Autodesk Fusion 360 part; units mm, degrees
(part 2 of 2)
  line L917 (-904.3735, -2837.0745) -> (-14000, -2837.0745)
  line L918 (-1204.3735, -11252.1545) -> (-1204.3735, -3137.0745)
  line L919 (-1204.3735, -3137.0745) -> (-14000, -3137.0745)
  line L920 (-14000, -3137.0745) -> (-14000, -2837.0745)
  line L921 (-1204.3735, -11252.1545) -> (-904.3735, -11252.1545)
  line L922 (-7006.0828, -10336.1218) -> (-8698.4144, -10336.1218)
  line L923 (-8698.4144, -10336.1218) -> (-8698.4144, -3137.0745)
  line L924 (-8698.4144, -3137.0745) -> (-7006.0828, -3137.0745)
  line L925 (-7006.0828, -3137.0745) -> (-7006.0828, -10336.1218)
  line L926 (-5639.7967, -10336.1218) -> (-1204.3735, -10336.1218)
  line L927 (-1204.3735, -10336.1218) -> (-1204.3735, -10036.1218)
  line L928 (-1204.3735, -10036.1218) -> (-5639.7967, -10036.1218)
  line L929 (-5639.7967, -10036.1218) -> (-5639.7967, -10336.1218)
  line L930 (-14200, -10000) -> (-9900, -10000)
  line L931 (-9900, -10000) -> (-9900, -10300)
  line L932 (-9900, -10300) -> (-14200, -10300)
  line L933 (-14200, -10300) -> (-14200, -10000)
  line L934 (-1060.2048, -1766.9819) -> (-14240.8305, -1766.9819)
  line L935 (-14240.8305, 3555.5601) -> (-1060.2048, 3555.5601)
  line L936 (-1360.2048, -1466.9819) -> (-13940.8305, -1466.9819)
  line L937 (-13940.8305, 3255.5601) -> (-1360.2048, 3255.5601)
  line L938 (-8963.6202, 3255.5601) -> (-9263.6202, 3255.5601)
  line L939 (-9263.6202, 3255.5601) -> (-9263.6202, -1466.9819)
  line L940 (-9263.6202, -1466.9819) -> (-8963.6202, -1466.9819)
  line L941 (-8963.6202, -1466.9819) -> (-8963.6202, 3255.5601)
  line L942 (-13940.8305, 758.7969) -> (-9263.6202, 758.7969)
  line L943 (-9263.6202, 758.7969) -> (-9263.6202, 1058.7969)
  line L944 (-9263.6202, 1058.7969) -> (-13940.8305, 1058.7969)
  line L945 (-13940.8305, 1058.7969) -> (-13940.8305, 758.7969)
  line L946 (-13940.8305, 1674.4472) -> (-14240.8305, 1674.4472)
  line L947 (-14240.8305, 201.9825) -> (-13940.8305, 201.9825)
  line L948 (-13940.8305, 758.7969) -> (-13940.8305, 1058.7969)
  line L949 (-1360.2048, 2862.3179) -> (-1060.2048, 2862.3179)
  line L950 (-1060.2048, 1785.8101) -> (-1360.2048, 1785.8101)
  line L951 (-1060.2048, 3555.5601) -> (-1060.2048, 2862.3179)
  line L952 (-1060.2048, 1785.8101) -> (-1060.2048, -1766.9819)
  line L953 (-1360.2048, 3255.5601) -> (-1360.2048, 2862.3179)
  line L954 (-1360.2048, 1785.8101) -> (-1360.2048, -1466.9819)
  line L955 (-14240.8305, -1766.9819) -> (-14240.8305, 201.9825)
  line L956 (-14240.8305, 1674.4472) -> (-14240.8305, 3555.5601)
  line L957 (-13940.8305, 1674.4472) -> (-13940.8305, 3255.5601)
  line L958 (-13940.8305, -1466.9819) -> (-13940.8305, 201.9825)
  line L959 (-13940.8305, 758.7969) -> (-13940.8305, 1058.7969)
  line L960 (-14240.8305, 3555.5601) -> (-13940.8305, 3555.5601)
  line L961 (-13940.8305, 3555.5601) -> (-13940.8305, 6300)
  line L962 (-13940.8305, 6300) -> (-14240.8305, 6300)
  line L963 (-14240.8305, 6300) -> (-14240.8305, 3555.5601)
  line L964 (-13500, 6000) -> (-11400, 6000)
  line L965 (-11400, 6000) -> (-11400, 3555.5601)
  line L966 (-13500, 6300) -> (-11100, 6300)
  line L967 (-11100, 6300) -> (-11100, 3555.5601)
  line L968 (-13500, 6000) -> (-13500, 6300)
  line L969 (-10700, 6000) -> (-9300, 6000)
  line L970 (-9300, 6000) -> (-9300, 3555.5601)
  line L971 (-10700, 6300) -> (-9000, 6300)
  line L972 (-9000, 6300) -> (-9000, 3555.5601)
  line L973 (-10700, 6300) -> (-10700, 6000)
  line L974 (-14200, 10200) -> (-9100, 10200)
  line L975 (-9100, 10200) -> (-9100, 7400)
  line L976 (-14200, 7400) -> (-14200, 10200)
  line L977 (-13900, 7700) -> (-13900, 9900)
  line L978 (-13900, 9900) -> (-9400, 9900)
  line L979 (-9400, 9900) -> (-9400, 7700)
  line L980 (-12500, 7700) -> (-12500, 7400)
  line L981 (-12000, 7400) -> (-12000, 7700)
  line L982 (-9800, 7700) -> (-9800, 7400)
  line L983 (-9400, 7400) -> (-9400, 7700)
  line L984 (-12000, 9900) -> (-11700, 9900)
  line L985 (-11700, 9900) -> (-11700, 7700)
  line L986 (-11700, 7700) -> (-12000, 7700)
  line L987 (-12000, 7700) -> (-12000, 9900)
  line L988 (-12500, 7400) -> (-14200, 7400)
  line L989 (-9800, 7700) -> (-12000, 7700)
  line L990 (-12500, 7700) -> (-13900, 7700)
  line L991 (-9100, 7400) -> (-9400, 7400)
  line L992 (-9800, 7400) -> (-12000, 7400)
  line L993 (-12500, 12200) -> (-13900, 12200)
  line L994 (-13900, 12200) -> (-13900, 14100)
  line L995 (-13900, 14100) -> (-12100, 14100)
  line L996 (-12100, 14100) -> (-12100, 12100)
  line L997 (-12500, 11900) -> (-14200, 11900)
  line L998 (-14200, 11900) -> (-14200, 14400)
  line L999 (-14200, 14400) -> (-11800, 14400)
  line L1000 (-11800, 14400) -> (-11800, 12200)
  line L1001 (-12500, 12200) -> (-12500, 11900)
  line L1002 (-12100, 12100) -> (-12100, 11900)
  line L1003 (-12100, 11900) -> (-9800, 11900)
  line L1004 (-9800, 11900) -> (-9800, 12200)
  line L1005 (-9800, 12200) -> (-11800, 12200)
  line L1006 (-11800, 14100) -> (-9400, 14100)
  line L1007 (-9400, 14100) -> (-9400, 12100)
  line L1008 (-9400, 12100) -> (-9100, 12100)
  line L1009 (-9100, 12100) -> (-9100, 14100)
  line L1010 (-11800, 14400) -> (-1049.606, 14400)
  line L1011 (-1049.606, 14400) -> (-1060.2048, 3555.5601)
  line L1012 (-9100, 14100) -> (-1595.3922, 14100)
  line L1013 (-1360.2048, 3555.5601) -> (-1360.2048, 14100)
  line L1014 (-1360.2048, 14100) -> (-1595.3922, 14100)
  line L1015 (-39100, 9500) -> (-31300, 9500)
  line L1016 (-31300, 9500) -> (-31300, 14500)
  line L1017 (-31300, 14500) -> (-27900, 14500)
  line L1018 (-39100, 9200) -> (-31000, 9200)
  line L1019 (-31000, 9200) -> (-31000, 14200)
  line L1020 (-31000, 14200) -> (-27900, 14200)
  line L1021 (-27900, 14500) -> (-27900, 14200)
  line L1022 (-31000, 9500) -> (-22000, 9500)
  line L1023 (-22000, 9500) -> (-22000, 14000)
  line L1024 (-22000, 14000) -> (-25200, 14000)
  line L1025 (-31000, 9200) -> (-21700, 9200)
  line L1026 (-21700, 9200) -> (-21700, 14300)
  line L1027 (-21700, 14300) -> (-25200, 14300)
  line L1028 (-25200, 14300) -> (-25200, 14000)
  line L1029 (-21700, 14300) -> (-18691.9492, 14300)
  line L1030 (-18691.9492, 14300) -> (-18691.9492, 14000)
  line L1031 (-18691.9492, 14000) -> (-21700, 14000)
  line L1032 (-26700, 14400) -> (-26400, 14400)
  line L1033 (-26400, 14400) -> (-26400, 9500)
  line L1034 (-26400, 9500) -> (-26700, 9500)
  line L1035 (-26700, 9500) -> (-26700, 14400)
  line L1036 (-21700, 9200) -> (-17491.9492, 9200)
  line L1037 (-17491.9492, 9200) -> (-17491.9492, 8300)
  line L1038 (-17491.9492, 8300) -> (-17191.9492, 8300)
  line L1039 (-17191.9492, 8300) -> (-17191.9492, 14200)
  line L1040 (-17191.9492, 9500) -> (-17191.9492, 8600)
  line L1041 (-21700, 9500) -> (-17491.9492, 9500)
  line L1042 (-17491.9492, 9500) -> (-17491.9492, 14200)
  line L1043 (-17491.9492, 14200) -> (-17191.9492, 14200)
  line L1044 (-31410.3645, 9200) -> (-31410.3645, 3640.3591)
  line L1045 (-31410.3645, 3640.3591) -> (-17160.8557, 3640.3591)
  line L1046 (-17160.8557, 3640.3591) -> (-17160.8557, 6838.9487)
  line L1047 (-31110.3645, 9200) -> (-31110.3645, 3940.3591)
  line L1048 (-31110.3645, 3940.3591) -> (-17460.8557, 3940.3591)
  line L1049 (-17460.8557, 3940.3591) -> (-17460.8557, 6838.9487)
  line L1050 (-17160.8557, 6838.9487) -> (-17460.8557, 6838.9487)
  line L1051 (15034.8266, -18499.5167) -> (15034.8266, -18199.5167)
  dimension "d1" = 90
  dimension "d4" = 90
  dimension "d13" = 90
  dimension "d24" = 90
  dimension "d25" = 90
  dimension "d68" = 90
  dimension "d101" = 90
  constraint horizontal L0
  constraint perpendicular L1 L2
  constraint perpendicular L2 L3
  constraint perpendicular L3 L4
  constraint perpendicular L2 L5
  constraint perpendicular L5 L6
  constraint perpendicular L6 L7
  constraint perpendicular L0 L16
  constraint perpendicular L16 L17
  constraint perpendicular L17 L18
  constraint perpendicular L18 L19
  constraint perpendicular L19 L20
  constraint perpendicular L18 L21
  constraint perpendicular L21 L22
  constraint perpendicular L22 L23
  constraint vertical L24
  constraint perpendicular L25 L26
  constraint perpendicular L26 L27
  constraint perpendicular L25 L28
  constraint perpendicular L28 L29
  constraint perpendicular L29 L30
  constraint vertical L52
  constraint coincident L38 L52.end
  constraint coincident L38 L53.start
  constraint perpendicular L38 L53
  constraint parallel L18 L31
  constraint parallel L22 L32
  constraint parallel L30 L33
  constraint parallel L29 L34
  constraint parallel L27 L35
  constraint parallel L26 L36
  constraint parallel L25 L37
  constraint parallel L24 L38
  constraint parallel L21 L39
  constraint parallel L20 L40
  constraint parallel L19 L41
  constraint parallel L16 L42
  constraint parallel L0 L43
  constraint parallel L1 L44
  constraint parallel L2 L45
  constraint parallel L3 L46
  constraint parallel L4 L47
  constraint parallel L5 L48
  constraint parallel L6 L49
  constraint parallel L7 L50
  constraint horizontal L55
  constraint vertical L56
  constraint horizontal L57
  constraint vertical L58
  constraint coincident L38 L55.start
  constraint horizontal L59
  constraint vertical L60
  constraint horizontal L61
  constraint vertical L62
  constraint coincident L36 L60.end
  constraint perpendicular L63 L66
  constraint perpendicular L66 L67
  constraint coincident L63 L68.end
  constraint perpendicular L63 L68
  constraint horizontal L69
  constraint vertical L70
  constraint horizontal L71
  constraint vertical L72
  constraint coincident L38 L70.end
  constraint coincident L38 L73.start
  constraint perpendicular L38 L73
  constraint perpendicular L73 L74
  constraint perpendicular L38 L75
  constraint perpendicular L75 L76
  constraint perpendicular L76 L80
  constraint coincident L36 L81.start
  constraint perpendicular L36 L81
  constraint perpendicular L81 L82
  constraint perpendicular L36 L83
  constraint perpendicular L84 L85
  constraint perpendicular L85 L89
  constraint perpendicular L35 L90
  constraint perpendicular L36 L91
  constraint perpendicular L35 L92
  constraint perpendicular L36 L93
  constraint perpendicular L93 L94
  constraint perpendicular L93 L95
  constraint perpendicular L36 L96
  constraint coincident L35 L97.end
  constraint perpendicular L35 L97
  constraint horizontal L98
  constraint vertical L99
  constraint horizontal L100
  constraint vertical L101
  constraint coincident L35 L102.start
  constraint perpendicular L35 L102
  constraint perpendicular L102 L103
  constraint perpendicular L103 L104
  constraint perpendicular L104 L105
  constraint horizontal L110
  constraint vertical L111
  constraint horizontal L112
  constraint vertical L113
  constraint coincident L35 L111.end
  constraint coincident L35 L114.start
  constraint perpendicular L35 L114
  constraint perpendicular L114 L115
  constraint perpendicular L35 L116
  constraint perpendicular L116 L117
  constraint perpendicular L117 L121
  constraint horizontal L122
  constraint vertical L123
  constraint horizontal L124
  constraint vertical L125
  constraint coincident L35 L123.end
  constraint perpendicular L35 L126
  constraint perpendicular L35 L128
  constraint perpendicular L35 L130
  constraint parallel L134 L136
  constraint perpendicular L134 L137
  constraint perpendicular L137 L138
  constraint perpendicular L134 L139
  constraint perpendicular L139 L140
  constraint perpendicular L140 L141
  constraint perpendicular L141 L142
  constraint perpendicular L142 L143
  constraint perpendicular L143 L144
  constraint perpendicular L144 L145
  constraint perpendicular L145 L146
  constraint perpendicular L146 L147
  constraint perpendicular L34 L148
  constraint perpendicular L148 L149
  constraint vertical L150
  constraint perpendicular L150 L151
  constraint perpendicular L153 L154
  constraint perpendicular L154 L155
  constraint perpendicular L155 L156
  constraint perpendicular L164 L165
  constraint coincident L159 L166.end
  constraint perpendicular L159 L166
  constraint perpendicular L165 L167
  constraint perpendicular L167 L168
  constraint coincident L159 L169.end
  constraint perpendicular L159 L169
  constraint horizontal L170
  constraint vertical L171
  constraint horizontal L172
  constraint vertical L173
  constraint coincident L159 L171.end
  constraint vertical L174
  constraint perpendicular L174 L175
  constraint perpendicular L175 L178
  constraint horizontal L185
  constraint vertical L179
  constraint horizontal L180
  constraint vertical L181
  constraint vertical L182
  constraint horizontal L183
  constraint vertical L184
  constraint collinear L185 L186
  constraint coincident L160 L187.start
  constraint perpendicular L160 L187
  constraint perpendicular L187 L188
  constraint horizontal L192
  constraint vertical L193
  constraint horizontal L194
  constraint vertical L195
  constraint coincident L160 L193.end
  constraint coincident L160 L196.start
  constraint perpendicular L160 L196
  constraint perpendicular L196 L197
  constraint perpendicular L160 L198
  constraint perpendicular L198 L199
  constraint horizontal L204
  constraint vertical L205
  constraint horizontal L206
  constraint vertical L207
  constraint coincident L160 L205.end
  constraint coincident L160 L208.start
  constraint perpendicular L160 L208
  constraint perpendicular L208 L209
  constraint perpendicular L160 L210
  constraint perpendicular L210 L211
  constraint horizontal L216
  constraint vertical L217
  constraint horizontal L218
  constraint vertical L219
  constraint coincident L160 L220.start
  constraint perpendicular L160 L220
  constraint perpendicular L220 L221
  constraint perpendicular L221 L222
  constraint perpendicular L222 L223
  constraint perpendicular L223 L227
  constraint parallel L160 L228
  constraint coincident L160 L229.end
  constraint perpendicular L160 L229
  constraint horizontal L233
  constraint vertical L234
  constraint horizontal L235
  constraint vertical L236
  constraint coincident L160 L233.start
  constraint horizontal L237
  constraint vertical L238
  constraint horizontal L239
  constraint vertical L240
  constraint coincident L236 L237.start
  constraint vertical L241
  constraint coincident L236 L242.end
  constraint perpendicular L236 L242
  constraint perpendicular L241 L245
  constraint perpendicular L241 L246
  constraint perpendicular L246 L247
  constraint perpendicular L247 L248
  constraint perpendicular L248 L249
  constraint perpendicular L243 L250
  constraint vertical L255
  constraint coincident L253 L256.end
  constraint perpendicular L253 L256
  constraint perpendicular L246 L257
  constraint perpendicular L255 L260
  constraint parallel L211 L261
  constraint perpendicular L211 L262
  constraint perpendicular L262 L263
  constraint perpendicular L263 L264
  constraint coincident L258 L265.end
  constraint perpendicular L258 L265
  constraint perpendicular L267 L271
  constraint coincident L268 L272.end
  constraint perpendicular L268 L272
  constraint horizontal L276
  constraint perpendicular L276 L277
  constraint perpendicular L277 L278
  constraint perpendicular L272 L279
  constraint coincident L273 L280.end
  constraint perpendicular L273 L280
  constraint perpendicular L276 L285
  constraint perpendicular L285 L286
  constraint perpendicular L286 L287
  constraint coincident L283 L288.end
  constraint perpendicular L283 L288
  constraint equal L284 L290
  constraint coincident L289 L292.start
  constraint perpendicular L289 L292
  constraint perpendicular L288 L293
  constraint perpendicular L289 L294
  constraint perpendicular L289 L295
  constraint perpendicular L295 L296
  constraint perpendicular L292 L302
  constraint coincident L299 L303.end
  constraint perpendicular L299 L303
  constraint horizontal L304
  constraint vertical L305
  constraint horizontal L306
  constraint vertical L307
  constraint coincident L307 L308.end
  constraint perpendicular L307 L308
  constraint horizontal L309
  constraint vertical L310
  constraint horizontal L311
  constraint vertical L312
  constraint coincident L236 L310.end
  constraint coincident L307 L309.start
  constraint horizontal L313
  constraint vertical L314
  constraint horizontal L315
  constraint vertical L316
  constraint coincident L298 L314.end
  constraint coincident L309 L313.start
  constraint horizontal L317
  constraint vertical L318
  constraint horizontal L319
  constraint vertical L320
  constraint horizontal L321
  constraint vertical L322
  constraint horizontal L323
  constraint vertical L324
  constraint coincident L307 L321.start
  constraint perpendicular L322 L325
  constraint perpendicular L325 L326
  constraint perpendicular L326 L327
  constraint perpendicular L325 L328
  constraint perpendicular L328 L329
  constraint perpendicular L325 L330
  constraint perpendicular L328 L331
  constraint perpendicular L331 L339
  constraint horizontal L340
  constraint vertical L341
  constraint horizontal L342
  constraint vertical L343
  constraint coincident L318 L341.end
  constraint coincident L334 L340.start
  constraint horizontal L344
  constraint perpendicular L344 L345
  constraint perpendicular L344 L346
  constraint perpendicular L346 L350
  constraint perpendicular L346 L351
  constraint coincident L347 L352.end
  constraint perpendicular L347 L352
  constraint perpendicular L351 L355
  constraint perpendicular L351 L356
  constraint coincident L354 L357.end
  constraint perpendicular L354 L357
  constraint horizontal L361
  constraint vertical L362
  constraint horizontal L363
  constraint vertical L364
  constraint coincident L236 L365.end
  constraint perpendicular L236 L365
  constraint perpendicular L236 L366
  constraint coincident L236 L366.end
  constraint horizontal L367
  constraint vertical L368
  constraint horizontal L369
  constraint vertical L370
  constraint coincident L371 L375.start
  constraint coincident L363 L375.end
  constraint perpendicular L363 L375
  constraint coincident L363 L376.end
  constraint perpendicular L363 L376
  constraint coincident L372 L377.start
  constraint perpendicular L372 L377
  constraint perpendicular L236 L378
  constraint perpendicular L378 L379
  constraint perpendicular L373 L380
  constraint perpendicular L372 L381
  constraint perpendicular L380 L382
  constraint coincident L374 L383.start
  constraint perpendicular L374 L383
  constraint perpendicular L383 L384
  constraint perpendicular L384 L387
  constraint coincident L385 L388.end
  constraint perpendicular L385 L388
  constraint perpendicular L388 L389
  constraint perpendicular L385 L390
  constraint horizontal L391
  constraint vertical L392
  constraint horizontal L393
  constraint vertical L394
  constraint horizontal L395
  constraint vertical L396
  constraint horizontal L397
  constraint vertical L398
  constraint coincident L392 L395.start
  constraint horizontal L399
  constraint vertical L400
  constraint horizontal L401
  constraint vertical L402
  constraint coincident L381 L403.start
  constraint perpendicular L381 L403
  constraint perpendicular L401 L404
  constraint perpendicular L400 L405
  constraint coincident L381 L408.end
  constraint perpendicular L381 L408
  constraint perpendicular L405 L409
  constraint horizontal L410
  constraint vertical L411
  constraint horizontal L412
  constraint vertical L413
  constraint parallel L336 L414
  constraint perpendicular L336 L415
  constraint coincident L373 L416.end
  constraint perpendicular L373 L416
  constraint perpendicular L414 L420
  constraint horizontal L421
  constraint vertical L422
  constraint horizontal L423
  constraint vertical L424
  constraint horizontal L440
  constraint vertical L425
  constraint horizontal L426
  constraint vertical L427
  constraint vertical L431
  constraint vertical L432
  constraint coincident L431.end L439
  constraint horizontal L433
  constraint vertical L434
  constraint horizontal L435
  constraint vertical L436
  constraint coincident L433.start L439
  constraint vertical L437
  constraint vertical L438
  constraint coincident L437.end L439
  constraint coincident L438.end L440
  constraint parallel L426 L428
  constraint parallel L427 L429
  constraint parallel L439 L440
  constraint parallel L425 L430
  constraint collinear L439 L443
  constraint collinear L440 L441
  constraint collinear L441 L442
  constraint collinear L443 L444
  constraint horizontal L445
  constraint vertical L446
  constraint horizontal L447
  constraint vertical L448
  constraint horizontal L449
  constraint coincident L342 L450.end
  constraint perpendicular L449 L453
  constraint perpendicular L452 L454
  constraint perpendicular L451 L455
  constraint coincident L452 L456.end
  constraint perpendicular L452 L456
  constraint coincident L335 L457.start
  constraint perpendicular L335 L457
  constraint perpendicular L330 L458
  constraint perpendicular L458 L461
  constraint coincident L318 L462.start
  constraint perpendicular L318 L462
  constraint coincident L318 L463.end
  constraint perpendicular L318 L463
  constraint perpendicular L463 L464
  constraint horizontal L465
  constraint perpendicular L465 L466
  constraint perpendicular L468 L469
  constraint perpendicular L469 L470
  constraint perpendicular L468 L471
  constraint perpendicular L471 L472
  constraint perpendicular L468 L473
  constraint perpendicular L466 L474
  constraint perpendicular L474 L475
  constraint perpendicular L320 L476
  constraint perpendicular L319 L477
  constraint perpendicular L319 L478
  constraint perpendicular L478 L479
  constraint perpendicular L478 L480
  constraint horizontal L481
  constraint vertical L482
  constraint horizontal L483
  constraint vertical L484
  constraint coincident L463 L481.start
  constraint horizontal L485
  constraint vertical L486
  constraint horizontal L487
  constraint vertical L488
  constraint horizontal L489
  constraint vertical L490
  constraint horizontal L491
  constraint vertical L492
  constraint horizontal L493
  constraint vertical L494
  constraint horizontal L495
  constraint vertical L496
  constraint coincident L492 L493.start
  constraint vertical L497
  constraint coincident L163 L498.end
  constraint perpendicular L163 L498
  constraint horizontal L501
  constraint vertical L502
  constraint horizontal L503
  constraint vertical L504
  constraint perpendicular L497 L505
  constraint vertical L506
  constraint coincident L488 L507.end
  constraint perpendicular L488 L507
  constraint horizontal L511
  constraint vertical L512
  constraint horizontal L513
  constraint vertical L514
  constraint coincident L509 L511.start
  constraint horizontal L515
  constraint vertical L516
  constraint horizontal L517
  constraint vertical L518
  constraint horizontal L519
  constraint vertical L520
  constraint horizontal L521
  constraint vertical L522
  constraint perpendicular L517 L523
  constraint perpendicular L518 L524
  constraint perpendicular L524 L527
  constraint perpendicular L524 L528
  constraint coincident L488 L529.end
  constraint perpendicular L488 L529
  constraint horizontal L531
  constraint vertical L532
  constraint horizontal L533
  constraint vertical L534
  constraint coincident L530 L532.end
  constraint horizontal L549
  constraint vertical L535
  constraint horizontal L536
  constraint vertical L537
  constraint vertical L541
  constraint vertical L542
  constraint coincident L542.end L549
  constraint vertical L543
  constraint vertical L544
  constraint parallel L536 L538
  constraint parallel L537 L539
  constraint parallel L547 L549
  constraint parallel L535 L540
  constraint collinear L545 L547
  constraint coincident L543.end L547
  constraint collinear L546 L549
  constraint collinear L547 L548
  constraint collinear L549 L550
  constraint horizontal L551
  constraint vertical L552
  constraint horizontal L553
  constraint vertical L554
  constraint coincident L548 L551.start
  constraint coincident L535 L555.start
  constraint perpendicular L535 L555
  constraint perpendicular L555 L556
  constraint perpendicular L535 L557
  constraint perpendicular L557 L558
  constraint perpendicular L535 L559
  constraint perpendicular L564 L566
  constraint perpendicular L565 L567
  constraint perpendicular L564 L568
  constraint perpendicular L565 L569
  constraint perpendicular L569 L570
  constraint perpendicular L565 L571
  constraint perpendicular L569 L572
  constraint perpendicular L572 L580
  constraint perpendicular L580 L581
  constraint parallel L579 L582
  constraint perpendicular L582 L583
  constraint perpendicular L583 L584
  constraint horizontal L585
  constraint coincident L581 L585.end
  constraint perpendicular L581 L585
  constraint perpendicular L584 L587
  constraint perpendicular L587 L588
  constraint perpendicular L588 L589
  constraint perpendicular L587 L590
  constraint perpendicular L50 L591
  constraint horizontal L592
  constraint coincident L587 L593.end
  constraint perpendicular L587 L593
  constraint perpendicular L595 L597
  constraint perpendicular L594 L598
  constraint coincident L595 L599.end
  constraint perpendicular L595 L599
  constraint horizontal L600
  constraint vertical L601
  constraint horizontal L602
  constraint vertical L603
  constraint coincident L587 L601.end
  constraint horizontal L604
  constraint parallel L587 L605
  constraint coincident L587 L606.end
  constraint perpendicular L587 L606
  constraint perpendicular L609 L611
  constraint perpendicular L608 L612
  constraint coincident L609 L613.end
  constraint perpendicular L609 L613
  constraint perpendicular L609 L614
  constraint perpendicular L608 L615
  constraint perpendicular L609 L616
  constraint coincident L587 L617.end
  constraint perpendicular L587 L617
  constraint perpendicular L614 L621
  constraint horizontal L622
  constraint vertical L623
  constraint horizontal L624
  constraint vertical L625
  constraint coincident L587 L623.end
  constraint horizontal L626
  constraint vertical L627
  constraint horizontal L628
  constraint vertical L629
  constraint horizontal L634
  constraint vertical L635
  constraint horizontal L636
  constraint vertical L637
  constraint horizontal L638
  constraint vertical L639
  constraint horizontal L640
  constraint vertical L641
  constraint perpendicular L639 L642
  constraint perpendicular L638 L643
  constraint perpendicular L643 L646
  constraint horizontal L648
  constraint vertical L649
  constraint horizontal L650
  constraint vertical L651
  constraint horizontal L652
  constraint vertical L653
  constraint horizontal L654
  constraint vertical L655
  constraint horizontal L656
  constraint vertical L657
  constraint horizontal L658
  constraint vertical L659
  constraint horizontal L660
  constraint vertical L661
  constraint horizontal L662
  constraint vertical L663
  constraint horizontal L664
  constraint vertical L665
  constraint horizontal L666
  constraint vertical L667
  constraint coincident L656 L668.start
  constraint perpendicular L656 L668
  constraint perpendicular L668 L669
  constraint perpendicular L656 L670
  constraint perpendicular L670 L671
  constraint perpendicular L671 L675
  constraint horizontal L676
  constraint perpendicular L676 L677
  constraint perpendicular L677 L678
  constraint perpendicular L678 L679
  constraint coincident L673 L680.end
  constraint perpendicular L676 L684
  constraint horizontal L685
  constraint vertical L686
  constraint horizontal L687
  constraint vertical L688
  constraint vertical L689
  constraint perpendicular L689 L690
  constraint perpendicular L690 L691
  constraint horizontal L697
  constraint vertical L698
  constraint horizontal L699
  constraint vertical L700
  constraint vertical L701
  constraint perpendicular L701 L702
  constraint perpendicular L702 L703
  constraint coincident L44 L704.end
  constraint perpendicular L44 L704
  constraint perpendicular L701 L708
  constraint horizontal L709
  constraint vertical L710
  constraint horizontal L711
  constraint vertical L712
  constraint vertical L713
  constraint perpendicular L713 L714
  constraint perpendicular L714 L715
  constraint coincident L44 L716.end
  constraint perpendicular L44 L716
  constraint horizontal L721
  constraint vertical L722
  constraint horizontal L723
  constraint vertical L724
  constraint vertical L725
  constraint perpendicular L725 L726
  constraint perpendicular L726 L727
  constraint coincident L44 L728.end
  constraint perpendicular L44 L728
  constraint perpendicular L725 L732
  constraint vertical L733
  constraint perpendicular L733 L734
  constraint perpendicular L733 L738
  constraint perpendicular L736 L739
  constraint perpendicular L733 L740
  constraint vertical L741
  constraint perpendicular L741 L742
  constraint perpendicular L742 L743
  constraint perpendicular L740 L747
  constraint coincident L745 L748.end
  constraint perpendicular L745 L748
  constraint perpendicular L741 L749
  constraint coincident L736 L754.end
  constraint perpendicular L736 L754
  constraint coincident L751 L755.start
  constraint coincident L736 L755.end
  constraint perpendicular L736 L755
  constraint perpendicular L739 L756
  constraint perpendicular L753 L757
  constraint perpendicular L743 L758
  constraint perpendicular L743 L759
  constraint perpendicular L758 L760
  constraint perpendicular L760 L761
  constraint perpendicular L762 L765
  constraint perpendicular L763 L766
  constraint perpendicular L766 L769
  constraint perpendicular L762 L770
  constraint perpendicular L770 L771
  constraint perpendicular L771 L772
  constraint perpendicular L772 L773
  constraint perpendicular L771 L774
  constraint perpendicular L774 L775
  constraint perpendicular L771 L776
  constraint perpendicular L776 L777
  constraint perpendicular L777 L778
  constraint perpendicular L774 L779
  constraint perpendicular L773 L780
  constraint perpendicular L778 L781
  constraint horizontal L782
  constraint vertical L783
  constraint horizontal L801
  constraint vertical L784
  constraint horizontal L789
  constraint vertical L790
  constraint horizontal L791
  constraint vertical L792
  constraint midpoint L788 L789.start
  constraint horizontal L793
  constraint vertical L794
  constraint horizontal L795
  constraint vertical L796
  constraint coincident L791 L793.start
  constraint vertical L797
  constraint vertical L798
  constraint coincident L797.end L801
  constraint vertical L799
  constraint vertical L800
  constraint coincident L799.end L801
  constraint collinear L801 L802
  constraint parallel L784 L786
  constraint parallel L782 L787
  constraint parallel L783 L788
  constraint collinear L802 L803
  constraint horizontal L830
  constraint vertical L804
  constraint horizontal L860
  constraint vertical L805
  constraint vertical L808
  constraint vertical L809
  constraint coincident L808.end L830
  constraint vertical L810
  constraint vertical L811
  constraint coincident L810.end L830
  constraint vertical L812
  constraint vertical L813
  constraint coincident L812.end L835
  constraint coincident L813.end L830
  constraint horizontal L814
  constraint vertical L815
  constraint coincident L815.end L830
  constraint vertical L816
  constraint vertical L817
  constraint coincident L816.end L860
  constraint vertical L818
  constraint vertical L819
  constraint coincident L818.end L860
  constraint vertical L820
  constraint vertical L821
  constraint collinear L822 L860
  constraint parallel L805 L806
  constraint parallel L830 L835
  constraint parallel L804 L807
  constraint horizontal L823
  constraint vertical L824
  constraint horizontal L825
  constraint vertical L826
  constraint parallel L823 L831
  constraint parallel L824 L827
  constraint parallel L825 L828
  constraint parallel L826 L829
  constraint collinear L830 L836
  constraint collinear L831 L832
  constraint coincident L807 L833.end
  constraint perpendicular L807 L833
  constraint coincident L827 L834.start
  constraint perpendicular L807 L834
  constraint collinear L835 L839
  constraint collinear L836 L837
  constraint collinear L837 L838
  constraint collinear L839 L840
  constraint coincident L807 L834.end
  constraint horizontal L841
  constraint vertical L842
  constraint horizontal L843
  constraint vertical L844
  constraint horizontal L845
  constraint vertical L846
  constraint horizontal L847
  constraint vertical L848
  constraint coincident L839 L845.start
  constraint horizontal L849
  constraint vertical L850
  constraint horizontal L851
  constraint vertical L852
  constraint horizontal L853
  constraint vertical L854
  constraint horizontal L855
  constraint vertical L856
  constraint coincident L854.end L858
  constraint coincident L833 L853.start
  constraint collinear L857 L860
  constraint collinear L858 L859
  constraint collinear L860 L861
  constraint horizontal L862
  constraint vertical L890
  constraint horizontal L863
  constraint vertical L888
  constraint horizontal L866
  constraint vertical L867
  constraint horizontal L868
  constraint vertical L869
  constraint coincident L865 L866.start
  constraint horizontal L870
  constraint vertical L871
  constraint horizontal L872
  constraint vertical L873
  constraint coincident L864 L871.end
  constraint horizontal L874
  constraint vertical L875
  constraint horizontal L876
  constraint vertical L877
  constraint horizontal L878
  constraint vertical L879
  constraint horizontal L880
  constraint vertical L881
  constraint horizontal L882
  constraint horizontal L883
  constraint coincident L882.start L888
  constraint horizontal L884
  constraint horizontal L885
  constraint coincident L885.start L890
  constraint parallel L863 L864
  constraint parallel L886 L888
  constraint parallel L862 L865
  constraint parallel L890 L892
  constraint collinear L886 L887
  constraint collinear L888 L889
  constraint collinear L890 L891
  constraint collinear L892 L893
  constraint horizontal L894
  constraint vertical L895
  constraint horizontal L896
  constraint vertical L897
  constraint horizontal L898
  constraint vertical L899
  constraint horizontal L900
  constraint vertical L901
  constraint vertical L902
  constraint perpendicular L902 L903
  constraint perpendicular L903 L904
  constraint perpendicular L904 L905
  constraint perpendicular L905 L910
  constraint horizontal L912
  constraint vertical L913
  constraint horizontal L914
  constraint vertical L915
  constraint vertical L916
  constraint perpendicular L916 L917
  constraint perpendicular L917 L920
  constraint perpendicular L916 L921
  constraint horizontal L922
  constraint vertical L923
  constraint horizontal L924
  constraint vertical L925
  constraint coincident L919 L923.end
  constraint horizontal L926
  constraint vertical L927
  constraint horizontal L928
  constraint vertical L929
  constraint horizontal L930
  constraint vertical L931
  constraint horizontal L932
  constraint vertical L933
  constraint horizontal L934
  constraint vertical L955
  constraint horizontal L935
  constraint vertical L951
  constraint horizontal L938
  constraint vertical L939
  constraint horizontal L940
  constraint vertical L941
  constraint coincident L937 L938.start
  constraint horizontal L942
  constraint vertical L943
  constraint horizontal L944
  constraint vertical L945
  constraint coincident L942.start L958
  constraint horizontal L946
  constraint horizontal L947
  constraint vertical L948
  constraint coincident L946.start L958
  constraint horizontal L949
  constraint horizontal L950
  constraint coincident L950.start L951
  constraint collinear L951 L952
  constraint parallel L934 L936
  constraint parallel L955 L958
  constraint parallel L935 L937
  constraint collinear L953 L954
  constraint collinear L955 L956
  constraint collinear L957 L958
  constraint collinear L958 L959
  constraint horizontal L960
  constraint vertical L961
  constraint horizontal L962
  constraint vertical L963
  constraint horizontal L964
  constraint coincident L935 L965.end
  constraint perpendicular L935 L965
  constraint perpendicular L968 L969
  constraint coincident L935 L970.end
  constraint perpendicular L935 L970
  constraint perpendicular L969 L973
  constraint horizontal L974
  constraint vertical L975
  constraint horizontal L991
  constraint vertical L976
  constraint vertical L980
  constraint vertical L981
  constraint coincident L980.end L991
  constraint vertical L982
  constraint vertical L983
  constraint coincident L982.end L991
  constraint horizontal L984
  constraint vertical L985
  constraint horizontal L986
  constraint vertical L987
  constraint coincident L978 L984.start
  constraint collinear L988 L991
  constraint parallel L976 L977
  constraint parallel L974 L978
  constraint parallel L975 L979
  constraint collinear L989 L990
  constraint collinear L991 L992
  constraint horizontal L993
  constraint perpendicular L993 L994
  constraint perpendicular L994 L995
  constraint perpendicular L995 L996
  constraint perpendicular L993 L1002
  constraint perpendicular L1002 L1003
  constraint perpendicular L993 L1004
  constraint perpendicular L1000 L1005
  constraint parallel L993 L997
  constraint parallel L994 L998
  constraint parallel L995 L999
  constraint parallel L996 L1000
  constraint coincident L1000 L1006.start
  constraint perpendicular L1000 L1006
  constraint perpendicular L995 L1007
  constraint perpendicular L1000 L1008
  constraint perpendicular L995 L1009
  constraint perpendicular L1000 L1010
  constraint perpendicular L1009 L1012
  constraint coincident L935 L1013.start
  constraint perpendicular L935 L1013
  constraint perpendicular L1013 L1014
  constraint perpendicular L40 L1015
  constraint perpendicular L39 L1016
  constraint perpendicular L40 L1017
  constraint perpendicular L1017 L1021
  constraint coincident L1019 L1022.start
  constraint perpendicular L1019 L1022
  constraint perpendicular L1015 L1023
  constraint perpendicular L1019 L1024
  constraint perpendicular L1024 L1028
  constraint perpendicular L1026 L1029
  constraint perpendicular L1027 L1030
  constraint coincident L1026 L1031.end
  constraint perpendicular L1026 L1031
  constraint horizontal L1032
  constraint vertical L1033
  constraint horizontal L1034
  constraint vertical L1035
  constraint perpendicular L1026 L1036
  constraint perpendicular L1025 L1037
  constraint perpendicular L1026 L1038
  constraint perpendicular L1025 L1039
  constraint perpendicular L1039 L1043
  constraint coincident L1018 L1044.start
  constraint perpendicular L1018 L1044
  constraint perpendicular L1044 L1045
  constraint perpendicular L1045 L1046
  constraint perpendicular L465 L1051
  measures "d1" angle of L0 L1
  measures "d4" angle of L24 L25
  measures "d13" angle of L83 L84
  measures "d24" angle of L151 L152
  measures "d25" angle of L152 L153
  measures "d68" angle of L449 L450
  measures "d101" angle of L679 L680
extrude "Extrude1" add sketch "Sketch1" along normal blind 3000 contours L0 L1 L2 L3 L4 L5 L6 L7 L8 L9 L10 L11 L12 L13 L14 L15 L16 L17 L18 L19 L20 L21 L22 L23 L24 L25 L26 L27 L28 L29 L30 L31 L32 L33 L34 L35 L36 L37 L38 L39 L40 L41 L42 L43 L44 L45 L46 L47 L48 L49 L50 L51 L52 L58 L60 L70 L100 L112 L124 L126 L127 L128 L129 L130 L131 L132 L133 L134 L135 L136 L137 L138 L139 L140 L141 L142 L143 L144 L145 L146 L147 L148 L149 L564 L566 L567 L568 L569 L570 L571 L572 L573 L574 L575 L576 L577 L578 L579 L580 L581 L582 L583 L584 L585 L586 L587 L588 L589 L590 L591 L602 L624 L655 L659 L665 L698 L710 L722 | L535 L555 L556 L557 L558 L559 L560 L561 L562 L563 L564 L565 L634 L648 | L562 L628 L634 L635 L636 L637 | L626 L627 L628 L629 L636 L641 | L560 L648 L649 L650 L651 | L627 L638 L639 L640 L641 | L535 L536 L537 L538 L539 L540 L542 L544 L545 L546 L547 L549 L553 | L587 L614 L615 L616 L617 L618 L619 L620 L621 | L538 L548 L551 L552 L553 L554 | L587 L622 L623 L624 L625 | L541 L543 L548 L550 L551 | L587 L604 L605 L606 L607 L608 L609 L610 | L609 L611 L612 L613 | L587 L600 L601 L602 L603 | L587 L592 L593 L594 L595 L596 | L595 L597 L598 L599 | L35 L122 L123 L124 L125 | L35 L114 L115 L116 L117 L118 L119 L120 L121 | L9 L44 L697 L698 L699 L700 | L35 L110 L111 L112 L113 | L9 L44 L701 L702 L703 L704 L705 L706 L707 L708 | L35 L102 L103 L104 L105 L106 L107 L108 L109 | L9 L44 L709 L710 L711 L712 | L35 L98 L99 L100 L101 | L9 L44 L713 L714 L715 L716 L717 L718 L719 L720 | L35 L90 L91 L92 L93 L94 L95 L96 L97 | L9 L44 L721 L722 L723 L724 | L36 L81 L82 L83 L84 L85 L86 L87 L88 L89 | L9 L44 L725 L726 L727 L728 L729 L730 L731 L732 | L36 L59 L60 L61 L62 | L9 L44 L664 L665 L666 L667 | L38 L55 L56 L57 L58 | L42 L656 L657 L658 L659 L662 | L656 L660 L661 L662 L663 | L38 L53 L54 L63 L64 L65 | L40 L652 L653 L654 L655 L685 | L656 L668 L669 L670 L671 L672 L673 L674 L675 | L652 L685 L686 L687 L688 | L38 L69 L70 L71 L72 | L63 L66 L67 L68 | L40 L1015 L1016 L1017 L1018 L1019 L1020 L1021 | L673 L676 L677 L678 L679 L680 L681 L682 L683 L684 | L1018 L1044 L1045 L1046 L1047 L1048 L1049 L1050 | L38 L73 L74 L75 L76 L77 L78 L79 L80 | L1019 L1022 L1023 L1024 L1025 L1026 L1027 L1028 L1034 | L1026 L1036 L1037 L1038 L1039 L1040 L1041 L1042 L1043 | L1022 L1032 L1033 L1034 L1035 | L1026 L1029 L1030 L1031 | L150 L151 L152 L153 L154 L155 L156 L157 L158 L159 L160 L161 L162 L163 L164 L171 L194 L206 L217 L218 L219 L233 L485 L489 L494 | L159 L165 L166 L167 L168 L169 | L159 L170 L171 L172 L173 | L485 L486 L487 L488 L520 | L159 L160 L172 L174 L175 L176 L177 L178 | L163 L497 L498 L499 L500 L501 L505 | L488 L506 L507 L508 L509 L510 L511 | L488 L528 L529 L530 L533 L534 | L500 L501 L502 L503 L504 | L530 L531 L532 L534 | L530 L533 L534 | L160 L187 L188 L189 L190 L191 | L163 L492 L493 L494 L495 L496 | L488 L516 L519 L520 L521 L522 | L509 L511 L512 L513 L514 | L160 L489 L490 L491 L492 L496 | L515 L516 L517 L518 L522 | L517 L523 L524 L525 L526 L527 | L160 L192 L193 L194 L195 | L160 L196 L197 L198 L199 L200 L201 L202 L203 | L160 L233 L234 L235 L236 L240 L310 | L160 L204 L205 L206 L207 | L160 L228 L229 L230 L231 L232 | L236 L237 L238 L239 L240 | L160 L208 L209 L210 L211 L212 L213 L214 L215 | L236 L362 L365 L366 | L160 L220 L221 L222 L223 L224 L225 L226 L227 | L236 L241 L242 L243 L244 L245 | L361 L362 L363 L364 | L160 L217 L218 L219 | L160 L216 L217 L219 | L236 L307 L309 L310 L311 L312 L313 | L363 L371 L375 L376 | L243 L246 L247 L248 L249 L250 L251 L252 L253 L254 L257 | L302 L304 L305 L306 L307 L312 L324 | L353 L358 L367 L368 L369 L370 L371 L372 L373 L374 | L298 L309 L313 L314 L315 L316 | L307 L321 L322 L323 L324 | L372 L377 L378 L379 L380 L381 L382 L391 | L289 L292 L293 L294 L295 L296 L297 L298 L299 L300 L301 L315 | L253 L255 L256 L258 L259 L260 | L299 L303 L307 L308 | L356 L358 L360 L371 | L354 L357 L358 L359 L367 L371 | L283 L286 L287 L288 L289 L290 L291 | L373 L414 L415 L416 L417 L418 L419 L420 L424 | L381 L400 L403 L404 L405 L406 L407 L408 L409 L422 | L273 L276 L277 L278 L279 L280 L281 L282 L283 L284 L285 | L258 L261 L262 L263 L264 L265 L266 L267 L268 L269 L270 | L352 L353 L354 L370 L371 L374 | L347 L352 L354 L371 | L406 L419 L421 L422 L423 L424 | L268 L271 L272 L273 L274 L275 | L344 L345 L346 L347 L348 L349 L350 | L374 L383 L384 L385 L386 L387 | L381 L391 L392 L393 L394 L398 L413 | L399 L400 L401 L402 | L351 L353 L355 L374 | L385 L388 L389 L390 | L392 L395 L396 L397 L398 | L392 L410 L411 L412 L413 | L317 L318 L319 L320 L341 L446 | L318 L334 L340 L341 L342 L343 | L325 L326 L327 L328 L329 L330 L331 L332 L333 L334 L335 L336 L337 L338 L339 L343 | L318 L462 L463 L464 L481 | L318 L445 L446 L447 L448 | L342 L449 L450 L451 L452 L453 | L463 L473 L479 L481 L482 L483 L484 | L335 L457 L458 L459 L460 L461 | L465 L466 L467 L468 L469 L470 L471 L472 L473 L474 L475 L476 L477 L478 L479 L480 L483 L1051 | L452 L454 L455 L456 | L425 L426 L427 L428 L429 L430 L432 L435 L437 L439 L440 L442 L444 | L428 L433 L434 L435 L436 L443 | L431 L433 L438 L441 L443 | L642 L643 L644 L645 L646 L647 | L689 L690 L691 L692 L693 L694 L695 L696 | L733 L734 L735 L736 L737 L738 | L736 L751 L754 L755 | L739 L740 L745 L747 L748 L750 L751 L752 L753 L756 L757 | L741 L742 L743 L744 L745 L746 L749 L758 | L758 L759 L760 L761 L762 L763 L764 L770 L771 L772 L773 L774 L775 L776 L777 L778 L779 L780 L781 | L762 L765 L766 L767 L768 L769 | L782 L783 L784 L786 L787 L788 L790 L792 L798 L800 L801 L803 | L786 L788 L789 L790 L791 L792 L793 | L785 L791 L793 L794 L795 L796 | L785 L795 L797 L799 L802 | L804 L807 L814 L817 L860 | L807 L827 L833 L834 L843 L847 L849 L853 | L834 L840 L841 L842 L843 L844 | L833 L853 L854 L855 L856 L858 | L812 L815 L838 L840 L841 | L816 L819 L855 L858 L861 | L834 L839 L845 L846 L847 L848 | L833 L849 L850 L851 L852 L859 | L810 L813 L837 L839 L845 | L806 L824 L825 L827 L828 L835 | L818 L820 L851 L857 L859 | L805 L806 L809 L826 L828 L829 L830 L831 | L805 L806 L821 L822 L828 | L808 L823 L827 L832 L835 L836 | L811 L827 L835 L836 | L862 L865 L866 L875 L879 L882 L884 L887 L889 L890 L892 | L878 L879 L880 L881 L892 | L874 L875 L876 L877 L887 | L865 L866 L867 L868 L869 | L863 L864 L872 L883 L885 L886 L888 L891 L893 L897 L899 | L893 L894 L895 L896 L897 | L886 L898 L899 L900 L901 | L864 L870 L871 L872 L873 | L902 L903 L904 L905 L906 L907 L908 L909 L910 L911 L912 | L909 L912 L913 L914 L915 | L916 L917 L918 L919 L920 L921 L924 L927 | L918 L926 L927 L928 L929 | L919 L922 L923 L924 L925 | L930 L931 L932 L933 | L934 L936 L940 L947 L950 L952 L954 L955 L958 | L936 L937 L938 L939 L940 L941 L943 | L935 L937 L938 L946 L949 L951 L953 L956 L957 L960 | L939 L942 L943 L944 L945 L948 L959 | L935 L1000 L1006 L1007 L1008 L1009 L1010 L1011 L1012 L1013 L1014 | L935 L960 L961 L962 L963 | L935 L969 L970 L971 L972 L973 | L993 L994 L995 L996 L997 L998 L999 L1000 L1001 L1002 L1003 L1004 L1005 | L935 L964 L965 L966 L967 L968 | L974 L975 L976 L977 L978 L979 L980 L983 L984 L988 L990 L991 | L978 L984 L985 L986 L987 L989 | L981 L982 L986 L989 L992 makes body 1 at (34082.4394, 1000, 23000) makes body 2 at (-12500, 1000, -10200) makes body 3 at (-33666.0206, 1000, 23397.9233) makes body 4 at (-5269.5823, 1000, 2837.0745) makes body 5 at (13300, 1000, 23300) makes body 6 at (-16781.5459, 1000, 27437.5117) makes body 7 at (-12766.6667, 2000, 10000) makes body 8 at (-26666.6667, 1000, 1800) makes body 9 at (52486.2863, 0, 22416.8968) makes body 10 at (-26244.5893, 1000, 2500) makes body 11 at (22700, 1000, 25000) makes body 12 at (-5453.7467, 1000, 1766.9819) makes body 13 at (-10106.0035, 1000, 21446.3937) makes body 14 at (-21989.1787, 1000, 21548.9807) makes body 15 at (-40400, 2000, 18900) makes body 16 at (-8733.3333, 0, 35712.22)
sketch "Sketch2" plane through (0, 0, 0) normal (0, 1, 0) x (1, 0, 0)
  line L0 (-50000, 49000) -> (54000, 49000)
  line L1 (54000, 49000) -> (54000, -40000)
  line L2 (54000, -40000) -> (-50000, -40000)
  line L3 (-50000, -40000) -> (-50000, 49000)
  constraint horizontal L0
  constraint vertical L1
  constraint horizontal L2
  constraint vertical L3
extrude "Extrude2" add sketch "Sketch2" against normal blind 1000 bodies 1 2 3 4 5 6 7 8 9 10 11 12 13 14 15 16
